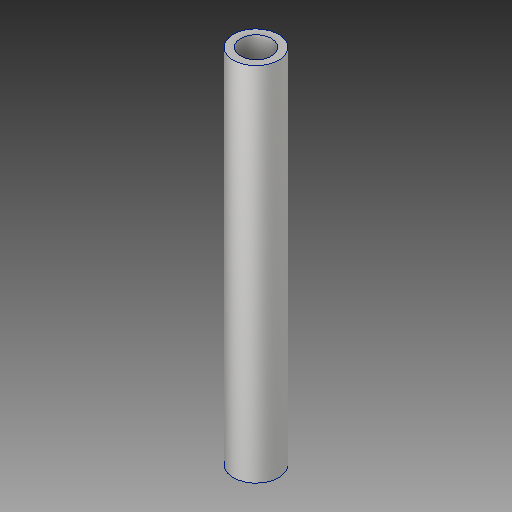
# Autodesk Inventor part: 1.25 Inch StandOff
Saved by Autodesk Inventor 2017 (Build 210142000, 142)
## iProperties
Created: 2018-01-26
Part Number: 1.25 Inch StandOff
Material: Aluminum 6061
Document SubType Name: Modeling
Designer: S346795925
Density: 2.7 g/cm^3
Appearance: Aluminum - Flat
Author: S346795925
Autodesk Inventor part; units mm, degrees
ref_plane "YZ Plane" through (0, 0, 0) normal (1, 0, 0) x (0, 1, 0)
ref_plane "XZ Plane" through (0, 0, 0) normal (0, 1, 0) x (-1, 0, 0)
ref_plane "XY Plane" through (0, 0, 0) normal (0, 0, 1) x (1, 0, 0)
sketch "Sketch1" plane through (0, 0, 0) normal (0, 1, 0) x (-1, 0, 0)
  circle A0 centre (0, 0) radius 3.175
  circle A1 centre (0, 0) radius 2.159
  dimension "d0" = 6.35
  dimension "d1" = 1.016
  constraints: 2 centre point, 1 coincident
  measures "d0" diameter of A0
  measures "d1" radial gap between concentric circles of A0 A1
extrude "Extrusion1" add sketch "Sketch1" along normal blind 50.8
body "Solid1"
